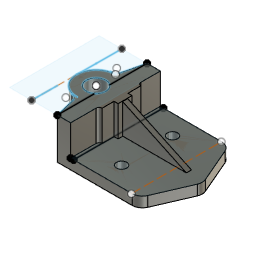
A3 (Autodesk Fusion 360 design; units mm, degrees)
Autodesk Fusion 360 part; units mm, degrees
note: some values were not read from the file. Set by a fixed rule: which sketch regions a step uses.
sketch "Sketch1" plane through (0, 0, 0) normal (0, 0, 1) x (1, 0, 0)
  line L0 (26.9257, 44) -> (-33.5, 44)
  line L1 (-33.5, 44) -> (-33.5, -44)
  line L2 (-33.5, -44) -> (26.9257, -44)
  line L3 (33.5, -44) -> (33.5, 44)
  line L4 (33.5, 44) -> (-33.5, -44) construction
  line L5 (-33.5, 44) -> (33.5, -44) construction
  line L6 (-2.5, 44) -> (-2.5, -44) construction
  line L7 (33.5, 25) -> (-33.5, 25) construction
  line L8 (33.5, -25) -> (-33.5, -25) construction
  circle A0 centre (-2.5, 25) radius 5
  circle A1 centre (-2.5, -25) radius 5
  line L9 (36.1063, 37.9644) -> (50.7881, 3.9644)
  line L10 (36.1063, -37.9644) -> (50.7881, -3.9644)
  arc A2 (50.7881, -3.9644) -> (50.7881, 3.9644) centre (41.6075, 0) ccw
  arc A3 (26.9257, -44) -> (36.1063, -37.9644) centre (26.9257, -34) ccw
  arc A4 (36.1063, 37.9644) -> (26.9257, 44) centre (26.9257, 34) ccw
  dimension "d1" = 67
  dimension "d2" = 88
  dimension "d3" = 31
  dimension "d4" = 19
  dimension "d5" = 50
  dimension "d6" = 10
  dimension "d7" = 10
  dimension "d9" = 10
  constraint horizontal L0
  constraint perpendicular L0 L1
  constraint parallel L0 L2
  constraint parallel L1 L3
  constraint coincident L4 origin
  constraint coincident L5 origin
  constraint coincident L0 L6.start
  constraint coincident L2 L6.end
  constraint perpendicular L2 L6
  constraint coincident L3 L7.start
  constraint coincident L1 L7.end
  constraint perpendicular L1 L7
  constraint coincident L3 L8.start
  constraint coincident L1 L8.end
  constraint perpendicular L1 L8
  constraint coincident L6 A0.centre
  constraint coincident L7 A0.centre
  constraint coincident L6 A1.centre
  constraint coincident L8 A1.centre
  constraint tangent L9 A2
  constraint tangent L10 A2
  constraint coincident L3.start L10
  constraint coincident L3.start L2
  constraint tangent L10 A3
  constraint tangent L2 A3
  constraint equal A2 A3
  constraint coincident L3.end L9
  constraint coincident L3.end L0
  constraint tangent L9 A4
  constraint tangent L0 A4
  constraint equal A2 A4
  measures "d1" distance of L1.end L3.start
  measures "d2" distance of L0.end L1.end
  measures "d3" distance of L1 L6
  measures "d4" distance of L0 L7
  measures "d5" distance of L7 L8
  measures "d6" diameter of A0
  measures "d7" diameter of A1
  measures "d9" radius of A2
extrude "Extrude1" add sketch "Sketch1" along normal blind 10 makes body 1
sketch "Sketch2" plane through (-33.5, 0, 0) normal (-1, 0, 0) x (0, -1, 0)
  line L0 (-44, 0) -> (44, 0)
  line L1 (44, 0) -> (44, 10)
  line L2 (44, 10) -> (-44, 10)
  line L3 (-44, 10) -> (-44, 0)
  line L4 (-44, 10) -> (44, 10)
  line L5 (44, 10) -> (44, 40)
  line L6 (44, 40) -> (-44, 40)
  line L7 (-44, 40) -> (-44, 10)
  dimension "d12" = 88
  dimension "d13" = 30
  constraint horizontal L4
  constraint vertical L5
  constraint horizontal L6
  constraint vertical L7
  constraint coincident L2.end L3.start
  measures "d12" distance of L2.end L1.end
  measures "d13" distance of L2.end L6.end
extrude "Extrude2" add sketch "Sketch2" along normal blind 60 contours L2 L4 L5 L6 L7 bodies 1
sketch "Sketch3" plane through (0, 0, 40) normal (0, 0, 1) x (-1, 0, 0)
  line L0 (33.5, 44) -> (33.5, -44)
  line L1 (33.5, -44) -> (93.5, -44)
  line L2 (93.5, -44) -> (93.5, 44)
  line L3 (93.5, 44) -> (33.5, 44)
  circle A0 centre (52.5, 0) radius 9.5
  line L4 (71.4996, -0.13) -> (71.4996, -0.13) construction
  line L5 (71.4996, -0.13) -> (71.8015, 44) construction
  line L6 (46.5, -44) -> (51.3961, -23.5998)
  line L7 (46.5, 44) -> (51.3961, 23.5998)
  line L8 (57.2304, -19) -> (52.5, -19)
  line L9 (57.2304, 19) -> (52.5, 19)
  arc A1 (57.2304, -19) -> (51.3961, -23.5998) centre (57.2304, -25) ccw
  arc A2 (51.3961, 23.5998) -> (57.2304, 19) centre (57.2304, 25) ccw
  arc A3 (52.5, -19) -> (52.5, 19) centre (52.5, 0) ccw
  line L10 (52.5, 19) -> (52.5, 21.309) construction
  line L11 (46.5, 44) -> (46.5, 7.3655)
  line L12 (46.5, -7.3655) -> (46.5, -44)
  line L13 (71.4996, -0.13) -> (71.3704, -19)
  line L14 (71.8015, 44) -> (71.6305, 19)
  line L15 (71.3704, -19) -> (71.1994, -44)
  arc A4 (71.4996, -0.13) -> (52.5, 19) centre (52.5, 0) ccw
  arc A5 (52.5, -19) -> (71.4996, -0.13) centre (52.5, 0) ccw
  dimension "d17" = 19
  dimension "d18" = 13
  dimension "d19" = 38
  dimension "d20" = 6
  dimension "d21" = 6
  dimension "d26" = 19
  dimension "d27" = 19
  constraint coincident L3 L7.start
  constraint coincident L1 L6.start
  constraint perpendicular L1 L11
  constraint concentric A0 A3
  constraint coincident L4.start A3
  constraint coincident L1 L15.end
  constraint coincident L3 L5.end
  constraint tangent L5 A3
  constraint tangent L8 A3
  constraint tangent L9 A3
  constraint tangent L8 A1
  constraint tangent L6 A1
  constraint tangent L9 A2
  constraint tangent L7 A2
  constraint coincident A2 L10.end
  constraint coincident A0 L11.end
  constraint coincident A0 L12.start
  constraint collinear L11 L12
  constraint coincident L5 L14.end
  constraint coincident L9 L14.end
  constraint coincident L8 L13.end
  constraint tangent L13 A4
  constraint tangent L9 A4
  constraint coincident L15.end L4
  constraint tangent L8 A5
  measures "d17" diameter of A0
  measures "d18" distance of L0 L11
  measures "d19" diameter of A3
  measures "d20" radius of A1
  measures "d21" radius of A2
  measures "d26" radius of A4
  measures "d4" radius of A5
extrude "Extrude5" cut sketch "Sketch3" against normal blind 40 contours L1 L2 L3 L7 L9 A2 A3 L13 L15 A4 bodies 1
extrude "Extrude4" cut sketch "Sketch3" against normal blind 40 contours A0 bodies 1
extrude "Extrude3" cut sketch "Sketch3" against normal blind 40 contours L1 L2 L3 L7 L9 A2 A3 L13 L15 A4 | L1 L6 L8 A1 A3 L13 L15 A5 bodies 1
extrude "Extrude6" add sketch "Sketch3" against normal blind 40 separate body contours L1 L6 L8 A1 A3 L13 L15 A5 makes body 2
extrude "Extrude7" cut sketch "Sketch3" against normal blind 40 contours L1 L6 L8 A1 A3 L13 L15 A5 bodies 2
sketch "Sketch4" plane through (-33.5, 0, 0) normal (-1, 0, 0) x (0, -1, 0)
  line L0 (-44, 0) -> (44, 0)
  line L1 (44, 0) -> (44, 10)
  line L2 (44, 10) -> (-44, 10)
  line L3 (-44, 10) -> (-44, 0)
extrude "Extrude8" add sketch "Sketch4" along normal blind 40 bodies 1 2
extrude "Extrude9" cut sketch "Sketch3" against normal blind 40 contours L1 L6 L8 A1 A3 L13 L15 A5 bodies 1
extrude "Extrude10" cut sketch "Sketch3" against normal blind 40 contours L1 L2 L3 L7 L9 A2 A3 L13 L15 A4 | A0 bodies 1
sketch "Sketch5" plane through (0, 0, 10) normal (0, 0, 1) x (-1, 0, 0)
  circle A0 centre (2.5, -25) radius 5
  circle A1 centre (2.5, 25) radius 5
  arc A2 (-36.1063, -37.9644) -> (-26.9257, -44) centre (-26.9257, -34) ccw
  line L0 (-26.9257, -44) -> (33.5, -44)
  line L1 (33.5, -44) -> (33.5, 44)
  line L2 (33.5, 44) -> (-26.9257, 44)
  arc A3 (-26.9257, 44) -> (-36.1063, 37.9644) centre (-26.9257, 34) ccw
  line L3 (-36.1063, 37.9644) -> (-50.7881, 3.9644)
  arc A4 (-50.7881, 3.9644) -> (-50.7881, -3.9644) centre (-41.6075, 0) ccw
  line L4 (-50.7881, -3.9644) -> (-36.1063, -37.9644)
  line L5 (30.5, 44) -> (30.5, -44) construction
  line L6 (30.5, 44) -> (33.5, 44) construction
  line L7 (30.5, 44) -> (30.5, -44)
  dimension "d40" = 3
  constraint coincident L2 L5.start
  constraint coincident L0 L5.end
  constraint perpendicular L0 L5
  constraint coincident L1.end L2.start
  constraint perpendicular L1 L6
  measures "d40" distance of L1 L5
sketch "Sketch6" plane through (-33.5, 0, 0) normal (1, 0, 0) x (0, 1, 0)
  line L0 (44, 10) -> (44, 40)
  line L1 (44, 40) -> (-44, 40)
  line L2 (-44, 40) -> (-44, 10)
  line L3 (-44, 10) -> (44, 10)
  line L4 (-16.0515, 40) -> (21.9485, 40)
  line L5 (21.9485, 40) -> (21.9485, 10)
  line L6 (21.9485, 10) -> (-16.0515, 10)
  line L7 (-16.0515, 10) -> (-16.0515, 40)
  dimension "d41" = 38
  constraint horizontal L4
  constraint vertical L5
  constraint horizontal L6
  constraint vertical L7
  constraint coincident L3 L5.end
  constraint coincident L1 L4.start
  measures "d41" distance of L4.start L4.end
extrude "Extrude11" add sketch "Sketch6" along normal blind 3 contours L1 L3 L4 L5 L6 L7 bodies 1
fillet "Fillet1" radius 3 1 edges at (-33.5, -16.0515, 25) on bodies 1
fillet "Fillet2" radius 3 1 edges at (-33.5, 21.9485, 25) on bodies 1
sketch "Sketch7" plane through (-30.5, 0, 0) normal (1, 0, 0) x (0, 1, 0)
  line L0 (-16.0515, 10) -> (21.9485, 10)
  line L1 (21.9485, 10) -> (21.9485, 40)
  line L2 (21.9485, 40) -> (-16.0515, 40)
  line L3 (-16.0515, 40) -> (-16.0515, 10)
  line L4 (-4.4258, 40) -> (9.2581, 40)
  line L5 (9.2581, 40) -> (9.2581, 10)
  line L6 (9.2581, 10) -> (-4.4258, 10)
  line L7 (-4.4258, 10) -> (-4.4258, 40)
  dimension "d48" = 13.6838
  constraint horizontal L4
  constraint vertical L5
  constraint horizontal L6
  constraint vertical L7
  constraint coincident L2 L4.start
  measures "d48" distance of L4.start L4.end
extrude "Extrude12" add sketch "Sketch7" along normal blind 4 contours L0 L2 L4 L5 L6 L7 bodies 1
sketch "Sketch8" plane through (0, 0, 10) normal (0, 0, 1) x (1, 0, 0)
sketch "Sketch9" plane through (0, 0, 0) normal (0, 1, 0) x (1, 0, 0)
  line L0 (-26.7848, -39.6904) -> (36.1082, -10.2175)
  line L1 (36.1082, -10.2175) -> (-26.7848, -10.2175)
  line L2 (-26.7848, -10.2175) -> (-26.7848, -39.6904)
  constraint horizontal L1
  constraint perpendicular L1 L2
sketch "Sketch10" plane through (0, 0, 10) normal (0, 0, 1) x (-1, 0, 0)
  line L0 (-26.6159, 44.5279) -> (-26.6159, -43.6768) construction
  constraint vertical L0
extrude "Extrude13" add sketch "Sketch9" along normal blind 5 bodies 1
